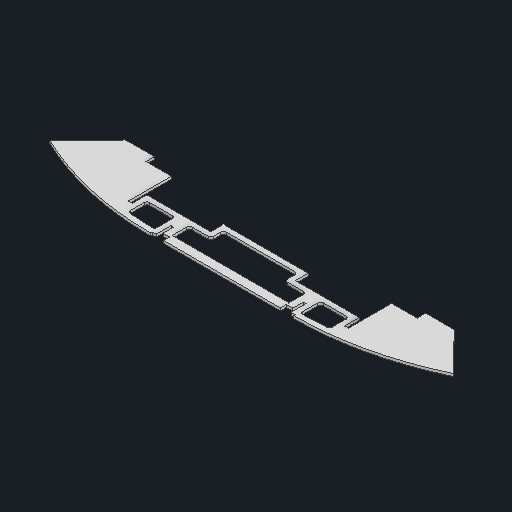
# Autodesk Inventor part: main
Saved by Autodesk Inventor 2023 (Build 270158030, 158C)
## iProperties
Created: 2022-03-21
Part Number: main
Material: Generic
Document SubType Name: Modeling
Designer: kardo
Density: 1 g/cm^3
Appearance: Default
Author: kardo
Autodesk Inventor part; units mm, degrees
ref_plane "YZ Plane" through (0, 0, 0) normal (1, 0, 0) x (0, 1, 0)
ref_plane "XZ Plane" through (0, 0, 0) normal (0, 1, 0) x (-1, 0, 0)
ref_plane "XY Plane" through (0, 0, 0) normal (0, 0, 1) x (1, 0, 0)
derived "parameters_frame.ipt"
derived "stencil_frame.ipt"
sketch "sk_joint_locations" plane through (81.12, 0, 0) normal (1, 0, 0) x (0, 1, 0)
  line L0 (0, 0) -> (111.39, 7.7891) construction
  line L1 (30.81, 28.832) -> (94.8, 28.832) construction
  arc A0 (30.81, 28.832) -> (9.48, 28.5282) centre (30.81, -720.1791) ccw construction
  line L2 (-254.1001, 21.0191) -> (9.48, 28.5282) construction
  line L3 (-363, 18.496) -> (-275.8801, 20.463) construction
  arc A1 (-275.8801, 20.463) -> (-254.1001, 21.0191) centre (-359.1231, 3707.4463) ccw construction
  line L4 (-210.8824, 4616.4994) -> (225.0382, -1617.4555) construction
  line L5 (-242.0001, 4592.9714) -> (-242.0001, -1605.7041) construction
  line L6 (-120.9999, 4592.9714) -> (-120.9999, -1605.7041) construction
  line L7 (-363, 4592.9714) -> (-363, -1605.7041) construction
  line L8 (0, 4592.9714) -> (0, -1605.7041) construction
  line L9 (551.8244, 47.4419) -> (-603.6686, 7.0912) construction
  line L10 (-657.8036, -26.1228) -> (709.4042, 69.4817) construction
  line L11 (178.2183, 30.3929) -> (177.9391, 38.388) construction
  line L12 (185.9231, 36.8959) -> (186.4825, 28.8959) construction
  line L13 (0, 6.528) -> (111.1168, 11.6964) construction
  line L14 (-242.0001, 45.8501) -> (-242.0001, 21.3638) construction
  line L15 (-363, 37.4293) -> (-363, 18.496) construction
  line L16 (-120.9999, 51.0063) -> (-120.9999, 24.811) construction
  line L17 (0, 52.89) -> (0, 28.2581) construction
  line L18 (108.3896, 50.6971) -> (108.935, 42.897) construction
  line L19 (109.4805, 35.0968) -> (108.935, 42.897) construction
  line L20 (109.4805, 35.0968) -> (110.0259, 27.2967) construction
  line L21 (110.0259, 27.2967) -> (110.5713, 19.4965) construction
  line L22 (110.5713, 19.4965) -> (111.1168, 11.6964) construction
  line L23 (0, 6.528) -> (0, 0) construction
  spline S0 degree 4 poles (-363, 37.4293) (-272.3626, 45.1427) (-181.5879, 49.7528) (-90.8131, 52.89) (0, 52.89) knots 0 0 0 0 0 1 1 1 1 1
  spline S1 degree 3 poles (0, 52.89) (86.3106, 52.89) (181.3207, 49.5034) (237, 36.448) knots 0 0 0 0 1 1 1 1
  spline S2 degree 2 poles (111.39, 7.7891) (176.0348, 12.3096) (237, 36.448) knots 0 0 0 1 1 1
  line L24 (94.8, 37.536) -> (94.8, 28.832) construction
  line L25 (94.8, 35.548) -> (94.8, 30.82) construction
  point P0 (-210.8824, 4616.4994)
  point P1 (225.0382, -1617.4555)
  point P2 (178.0787, 34.3904)
  point P3 (186.2028, 32.8959)
  point P4 (134.9575, 11.3411)
  point P5 (-363, 27.9627)
  point P6 (-242.0001, 33.6069)
  point P7 (-120.9999, 37.9086)
  point P8 (0, 40.5741)
  point P9 (94.8, 33.184)
sketch "sk_cowl_joint_locations" plane through (54.6, 0, 0) normal (1, 0, 0) x (0, 1, 0)
  line L0 (-363, 18.496) -> (-275.8801, 20.463) construction
  arc A0 (-275.8801, 20.463) -> (-254.1001, 21.0191) centre (-359.1231, 3707.4463) ccw construction
  line L1 (-254.1001, 21.0191) -> (9.48, 28.5282) construction
  arc A1 (30.81, 28.832) -> (9.48, 28.5282) centre (30.81, -720.1791) ccw construction
  line L2 (30.81, 28.832) -> (94.8, 28.832) construction
  line L3 (94.8, 30.032) -> (30.81, 30.032) construction
  arc A2 (30.81, 30.032) -> (9.4458, 29.7277) centre (30.81, -720.1791) ccw construction
  line L4 (9.4458, 29.7277) -> (-254.1343, 22.2186) construction
  arc A3 (-275.9072, 21.6626) -> (-254.1343, 22.2186) centre (-359.1231, 3707.4463) ccw construction
  line L5 (-275.9072, 21.6626) -> (-363, 19.6963) construction
  line L6 (-242.0001, 4592.9714) -> (-242.0001, -1605.7041) construction
  line L7 (-120.9999, 4592.9714) -> (-120.9999, -1605.7041) construction
  line L8 (-363, 4592.9714) -> (-363, -1605.7041) construction
  line L9 (0, 4592.9714) -> (0, -1605.7041) construction
  line L10 (-242.0001, 45.0688) -> (-242.0001, 22.5643) construction
  line L11 (-120.9999, 49.9661) -> (-120.9999, 26.0115) construction
  line L12 (-363, 19.6963) -> (-363, 19.6963)
  line L13 (-363, 19.6963) -> (-363, 36.9211) construction
  line L14 (-1229.7832, 4422.8213) -> (280.3081, -1633.8241) construction
  line L15 (-362.7741, 36.9211) -> (-363, 39.712) construction
  line L16 (0, 51.6) -> (0, 29.4586) construction
  spline S0 degree 2 poles (-363, 39.712) (-181.6483, 54.394) (0, 54.4) knots 0 0 0 1 1 1
  spline S1 degree 3 poles (0, 54.4) (31.284, 54.4) (68.256, 47.9917) (94.8, 37.536) knots 1 1 1 1 2 2 2 2
  spline S2 degree 3 poles (93.7738, 34.9308) (89.4268, 36.6431) (81.2968, 39.4556) (71.234, 42.2519) (63.4432, 44.1558) (58.1419, 45.3261) (51.4169, 46.6598) (45.9725, 47.6212) (39.1225, 48.6857) (33.6211, 49.4253) (26.7536, 50.2046) (21.2812, 50.7098) (14.5037, 51.1886) (7.8073, 51.5121) (2.5751, 51.6) (0, 51.6) knots 1 1 1 1 1.166667 1.291667 1.333333 1.416667 1.458333 1.541667 1.583333 1.666667 1.708333 1.791667 1.833333 1.916667 2 2 2 2
  spline S3 degree 3 poles (0, 51.6) (-20.1706, 51.5993) (-55.4643, 51.3605) (-95.7903, 50.6123) (-126.0307, 49.8474) (-146.1889, 49.2356) (-171.3841, 48.3435) (-191.5382, 47.528) (-216.7283, 46.3813) (-236.8783, 45.3621) (-262.0632, 43.9608) (-282.2091, 42.7379) (-307.3889, 41.082) (-332.5661, 39.2987) (-352.7052, 37.7363) (-362.7741, 36.9211) knots 0 0 0 0 0.166667 0.291667 0.333333 0.416667 0.458333 0.541667 0.583333 0.666666 0.708333 0.791666 0.833333 0.916666 1 1 1 1
  line L17 (-142.5135, 45.4866) -> (-137.5404, 25.5402) construction
  line L18 (-134.9025, 31.4945) -> (-138.7836, 30.5268) construction
  line L19 (-137.3891, 41.4677) -> (-141.2702, 40.5) construction
  line L20 (-142.5135, 45.4866) -> (-138.6324, 46.4543) construction
  line L21 (-137.5404, 25.5402) -> (-133.6592, 26.5079) construction
  line L22 (-138.6324, 46.4543) -> (-138.8117, 52.2515) construction
  point P0 (0, 0)
  point P1 (-363, 28.3087)
  point P2 (-242.0001, 33.8165)
  point P3 (-120.9999, 37.9888)
  point P4 (0, 40.5293)
  point P5 (-1229.7832, 4422.8213)
  point P6 (280.3081, -1633.8241)
  point P7 (-85.2629, 50.788)
  point P8 (0, 40.5293)
sketch "sk_main_base" plane through (0, 0, 0) normal (0, 1, 0) x (-1, 0, 0)
  line L0 (0, -1605.7041) -> (0, 4592.9714) construction
  line L1 (-81.12, 6.528) -> (-112.356, 43.7537) construction
  spline S0 degree 2 poles (-54.6, 54.4) (-107.2974, 54.4) (-156, 31.008) knots 0 0 0 1 1 1 construction
  line L2 (0, 54.4) -> (-54.6, 54.4) construction
  line L3 (0, 19.696) -> (-32.32, 19.696)
  line L4 (-32.32, 19.696) -> (-32.32, 29.4581)
  line L5 (-32.32, 29.4581) -> (-81.12, 29.4581)
  line L6 (-81.12, 40.5741) -> (-81.12, 29.4581)
  line L7 (-81.12, 40.5741) -> (-84.12, 40.5741)
  line L8 (-84.12, 40.5741) -> (-84.12, 7.728)
  line L9 (-125.5387, 1.2) -> (-153.978, 30.6419)
  line L10 (-54.6, 53.2) -> (0, 53.2)
  line L11 (0, 53.2) -> (0, 19.696)
  line L12 (-156, 31.008) -> (-126.048, 0) construction
  line L13 (-126.048, 0) -> (-81.12, 0) construction
  line L14 (-84.12, 7.728) -> (-103.584, 7.728)
  line L15 (-103.584, 7.728) -> (-103.584, 1.2)
  line L16 (-103.584, 1.2) -> (-125.5387, 1.2)
  line L17 (-103.584, 6.528) -> (-103.584, 0) construction
  spline S1 degree 5 poles (-155.4805, 29.9263) (-136.6548, 38.9668) (-116.9079, 46.0847) (-96.3691, 50.8985) (-75.4831, 53.1986) (-54.6, 53.2) knots 0 0 0 0 0 0 1 1 1 1 1 1
  point P0 (0, 0)
  point P1 (-34.32, 18.496)
  point P2 (-34.32, 28.2581)
  dimension "d3" = 1.2
  dimension "d5" = 3
  dimension "d6" = 1.2
  dimension "d7" = 1.2
  dimension "d8" = 2
  dimension "d11" = 1.2
  dimension "d12" = 1.2
  dimension "d13" = 1.2
  constraints: 24 end point, 6 parallel, 4 perpendicular, 2 collinear, 1 point on line, 4 other
  measures "d5" distance of L6.start L7.end
  measures "d6" distance from line of point (-34.32, 28.258) L5
  measures "d7" distance from line of L3 point (-34.32, 18.496)
  measures "d8" distance from line of L4 point (-34.32, 28.258)
  measures "d11" distance from line of L1.start L14
  measures "d12" distance between parallel lines of L13 L16
  measures "d13" distance between parallel lines of L12 L9
extrude "thicken" add sketch "sk_main_base" along normal blind 2
sketch "sk_stringer_cowl_cut" plane through (0, 0, 0) normal (0, 1, 0) x (-1, 0, 0)
  line L0 (-54.6, -1605.7041) -> (-54.6, 4592.9714) construction
  line L1 (-49.6, 90.5293) -> (-51.6, 90.5293)
  line L2 (-51.6, 90.5293) -> (-51.6, 40.5293)
  line L3 (-51.6, 40.5293) -> (-49.6, 40.5293)
  line L4 (-49.6, 40.5293) -> (-49.6, 90.5293)
  point P0 (0, 0)
  point P1 (-54.6, 40.5293)
  dimension "d14" = 5
  dimension "d15" = 2
  dimension "d20" = 50
  constraints: 8 end point, 3 parallel, 1 horizontal, 1 perpendicular, 1 point on line
  measures "d14" distance between parallel lines of L0 L4
  measures "d15" distance between parallel lines of L4 L2
  measures "d20" distance of L3.end L1.start
extrude "cut_joint" cut sketch "sk_stringer_cowl_cut" along normal through all both and the other way through all
sketch "sk_cowl_liner_cut" plane through (0, 0, 0) normal (0, 1, 0) x (-1, 0, 0)
  line L0 (0, 54.4) -> (-54.6, 54.4) projected
  line L1 (-54.6, 54.4) -> (-54.6, 52)
  line L2 (-54.6, 52) -> (-49.6, 52)
  line L3 (-49.6, 52) -> (-49.6, 48.6)
  line L4 (-49.6, 48.6) -> (-44.6, 48.6)
  line L5 (-44.6, 48.6) -> (-44.6, 54.4)
  point P0 (0, 0)
  dimension "d21" = 2.4
  dimension "d23" = 5
  dimension "d24" = 5
  dimension "d40" = 5.8
  constraints: 10 end point, 3 perpendicular, 2 parallel, 1 point on line
  measures "d21" distance between parallel lines of L0 L2
  measures "d23" distance of L1.end L2.end
  measures "d24" distance of L3.end L4.end
  measures "d40" distance of L4.end L5.end
extrude "cut_liner" cut sketch "sk_cowl_liner_cut" along normal through all both and the other way through all
sketch "sk_cut_weight" plane through (0, 0, 0) normal (0, 1, 0) x (-1, 0, 0)
  line L0 (0, 19.696) -> (-32.32, 19.696) construction
  line L1 (-32.32, 19.696) -> (-32.32, 29.4581) construction
  line L2 (-32.32, 29.4581) -> (-81.12, 29.4581) construction
  line L3 (-81.12, 40.5741) -> (-81.12, 29.4581) construction
  spline S0 degree 3 poles (-155.4805, 29.9263) (-152.7874, 31.2198) (-147.3834, 33.6987) (-140.5832, 36.5276) (-133.7491, 39.1542) (-128.2546, 41.0936) (-121.3525, 43.3158) (-115.8035, 44.9319) (-108.8331, 46.7498) (-103.2294, 48.0425) (-96.1903, 49.4564) (-90.5315, 50.426) (-83.4235, 51.4359) (-77.7094, 52.0823) (-70.532, 52.6882) (-63.3198, 53.0923) (-57.5128, 53.2) (-54.6, 53.2) knots 0 0 0 0 0.083333 0.166667 0.208333 0.291667 0.333333 0.416667 0.458333 0.541667 0.583333 0.666667 0.708333 0.791667 0.833333 0.916667 1 1 1 1 construction
  line L4 (-44.6, 48.6) -> (-44.6, 54.4) construction
  line L5 (-49.6, 48.6) -> (-44.6, 48.6) construction
  line L6 (-49.6, 52) -> (-49.6, 48.6) construction
  line L7 (0, -1605.7041) -> (0, 4592.9714) projected
  line L8 (0, 23.696) -> (-28.32, 23.696)
  line L9 (-28.32, 23.696) -> (-28.32, 33.4581)
  line L10 (-28.32, 33.4581) -> (-44.6, 33.4581)
  line L11 (-44.6, 33.4581) -> (-44.6, 46.6)
  line L12 (-44.6, 46.6) -> (0, 46.6)
  line L13 (-55.6, 49.2) -> (-55.6, 33.4581)
  line L14 (-55.6, 33.4581) -> (-77.12, 33.4581)
  line L15 (-77.12, 33.4581) -> (-77.12, 48.1087)
  line L16 (-77.12, 48.1087) -> (-55.6, 49.2)
  line L17 (-49.6, 29.4581) -> (-49.6, 48.6) construction
  line L18 (-51.6, 29.4581) -> (-51.6, 48.6) construction
  line L19 (-51.6, 48.6) -> (-49.6, 48.6) construction
  line L20 (-77.12, 48.1087) -> (-77.12, 52.1087) construction
  point P0 (0, 0)
  dimension "d27" = 2
  dimension "d28" = 4
  dimension "d29" = 4
  dimension "d30" = 4
  dimension "d31" = 4
  dimension "d32" = 4
  dimension "d33" = 4
  dimension "d34" = 4
  dimension "d35" = 4
  dimension "d36" = 2
  constraints: 26 end point, 9 parallel, 4 point on line, 3 collinear, 1 perpendicular, 1 other
  measures "d27" distance between parallel lines of L17 L18
  measures "d28" distance between parallel lines of L18 L13
  measures "d29" distance between parallel lines of L2 L14
  measures "d30" distance between parallel lines of L3 L15
  measures "d31" distance of L15.end L20.end
  measures "d32" vertical distance of point (-54.6, 53.2) L13.start
  measures "d33" distance between parallel lines of L2 L10
  measures "d34" distance between parallel lines of L1 L9
  measures "d35" distance between parallel lines of L0 L8
  measures "d36" distance between parallel lines of L12 L5
extrude "cut_weight" cut sketch "sk_cut_weight" along normal through all both and the other way through all
fillet "rounding" radius 2 7 edges at (77.12, 1, 33.4581) (28.32, 1, 23.696) (28.32, 1, 33.4581) (44.6, 1, 33.4581) (77.12, 1, 48.1087) (55.6, 1, 49.2) (55.6, 1, 33.4581)
mirror "mirror" about plane through (0, 0, 0) normal (1, 0, 0)
equation "\"d3\" = shell_thickness"
equation "\"d5\" = stringer_thickness"
equation "\"d6\" = shell_thickness"
equation "\"d7\" = shell_thickness"
equation "\"d8\" = bulkhead_thickness"
equation "\"d11\" = shell_thickness"
equation "\"d12\" = shell_thickness"
equation "\"d13\" = shell_thickness"
equation "\"d9\" = bulkhead_thickness"
equation "\"d14\" = cowl_liner_width"
equation "\"d15\" = bulkhead_thickness"
equation "\"d21\" = cowl_liner_thickness + shell_thickness"
equation "\"d23\" = cowl_liner_width"
equation "\"d24\" = cowl_sealing_width"
equation "\"d40\" = cowl_sealing_thickness + cowl_shell_thickness + cowl_liner_thickness"
equation "\"d27\" = bulkhead_thickness"
equation "\"d28\" = bulkhead_inset"
equation "\"d29\" = bulkhead_inset"
equation "\"d30\" = bulkhead_inset"
equation "\"d31\" = bulkhead_inset"
equation "\"d32\" = bulkhead_inset"
equation "\"d33\" = bulkhead_inset"
equation "\"d34\" = bulkhead_inset"
equation "\"d35\" = bulkhead_inset"
equation "\"shell_thickness\" = 1.2"
equation "\"stringer_thickness\" = 3"
equation "\"bulkhead_thickness\" = 2"
equation "\"cowl_liner_width\" = 5"
equation "\"cowl_liner_thickness\" = 1.2"
equation "\"cowl_sealing_width\" = 5"
equation "\"cowl_sealing_thickness\" = 3"
equation "\"cowl_shell_thickness\" = 1.6"
equation "\"bulkhead_inset\" = 4"
body "Solid1"
